robot-yaw-object-study-2026-10-04 (Autodesk Fusion 360 design; units mm, degrees)
Autodesk Fusion 360 part; units mm, degrees
sketch "Layout_Side" plane through (0, 0, 0) normal (0, 1, 0) x (1, 0, 0) in component "00_Layout"
  line L0 (0, 0) -> (0, -1676.4) construction
  line L1 (300, -275) -> (-300, -275) construction
  line L2 (-300, -275) -> (-300, -75) construction
  line L3 (-300, -75) -> (300, -75) construction
  line L4 (300, -75) -> (300, -275) construction
  line L5 (300, -275) -> (-300, -75) construction
  line L6 (-300, -275) -> (300, -75) construction
  line L7 (0, -1676.4) -> (600, -1676.4) construction
  line L8 (0, -175) -> (0, -75) construction
  dimension "d1" = 200
  dimension "d2" = 600
  dimension "d4" = 600
  dimension "d5" = 75
  dimension "d6" = 1676.4
  constraint vertical L0
  constraint horizontal L1
  constraint perpendicular L1 L2
  constraint parallel L1 L3
  constraint parallel L2 L4
  constraint perpendicular L0 L7
  constraint midpoint L3 L8.end
  constraint coincident L0.start origin
  constraint midpoint L8.start L5
  measures "d1" distance of L1.end L2.end
  measures "d2" distance of L1.start L1.end
  measures "d4" distance of L0.end L7.end
  measures "d5" distance of L0.start L8.end
  measures "d6" distance of L0.end L0.start
sketch "Base_Profile" plane through (0, 0, 0) normal (0, 1, 0) x (1, 0, 0) in component "01_Base_Envelope"
  line L0 (300, -275) -> (-300, -275)
  line L1 (-300, -275) -> (-300, -75)
  line L2 (-300, -75) -> (300, -75)
  line L3 (300, -75) -> (300, -275)
extrude "Chassis_Width_450mm" add sketch "Base_Profile" along normal mid plane 450 makes body 1 in component "01_Base_Envelope"
sketch "Mast_Envelope_Side_Profile" plane through (0, 0, 0) normal (0, 1, 0) x (1, 0, 0) in component "02_Mast_Envelope"
  line L0 (-160, -275) -> (-40, -275)
  line L1 (-40, -275) -> (-40, -1600)
  line L2 (-40, -1600) -> (-160, -1600)
  line L3 (-160, -1600) -> (-160, -275)
  line L4 (300, -275) -> (-300, -275) construction
  dimension "d9" = 120
  dimension "d10" = 1325
  dimension "d11" = 160
  constraint horizontal L0
  constraint vertical L1
  constraint horizontal L2
  constraint vertical L3
  constraint coincident L0.start L4
  measures "d9" horizontal distance of L0.start L0.end
  measures "d10" vertical distance of L0.end L1.end
  measures "d11" horizontal distance of origin L0.start
extrude "Mast_Envelope_Width_140mm" add sketch "Mast_Envelope_Side_Profile" along normal mid plane 140 separate body makes body 2 in component "02_Mast_Envelope"
sketch "Shared_Carriage_Side_Profile" plane through (0, 0, 0) normal (0, 1, 0) x (1, 0, 0) in component "03_Shared_Carriage"
  line L0 (-40, -840) -> (80, -840)
  line L1 (80, -840) -> (80, -960)
  line L2 (80, -960) -> (-40, -960)
  line L3 (-40, -960) -> (-40, -840)
  dimension "d14" = 120
  dimension "d15" = 120
  dimension "d16" = 40
  dimension "d17" = 840
  constraint horizontal L0
  constraint vertical L1
  constraint horizontal L2
  constraint vertical L3
  measures "d14" horizontal distance of L0.start L0.end
  measures "d15" vertical distance of L0.end L1.end
  measures "d16" horizontal distance of origin L0.start
  measures "d17" vertical distance of origin L0.start
extrude "Shared_Carriage_Width_660mm" add sketch "Shared_Carriage_Side_Profile" along normal mid plane 660 separate body makes body 3 in component "03_Shared_Carriage"
ref_plane "WorkPlane1" through (0, 300, 0) normal (0, 1, 0) x (0, 0, 1) in component "00_Layout"
sketch "Reach_Left_Floor_2x304p8mm" plane through (0, 300, 0) normal (0, 1, 0) x (1, 0, 0) in component "00_Layout"
  circle A0 centre (80, -400) radius 609.6 construction
  line L0 (80, -400) -> (380.0994, -346.6765) construction
  line L1 (380.0994, -346.6765) -> (450, -50) construction
  dimension "d25" = 80
  dimension "d26" = 400
  dimension "d27" = 450
  dimension "d28" = 50
  dimension "d29" = 609.6
  dimension "d30" = 304.8
  dimension "d31" = 304.8
  measures "d25" horizontal distance of origin A0.centre
  measures "d26" vertical distance of origin A0.centre
  measures "d27" horizontal distance of origin L1.end
  measures "d28" vertical distance of origin L1.end
  measures "d29" radius of A0
  measures "d30" distance of A0.centre L0.end
  measures "d31" distance of L1.end L0.end
sketch "Reach_Left_Shelf_2x304p8mm" plane through (0, 300, 0) normal (0, 1, 0) x (1, 0, 0) in component "00_Layout"
  circle A0 centre (80, -1400) radius 609.6 construction
  line L0 (80, -1400) -> (198.6357, -1680.7643) construction
  line L1 (198.6357, -1680.7643) -> (500, -1726.4) construction
  dimension "d32" = 80
  dimension "d33" = 1400
  dimension "d34" = 500
  dimension "d35" = 1726.4
  dimension "d36" = 609.6
  dimension "d37" = 304.8
  dimension "d38" = 304.8
  measures "d32" horizontal distance of origin A0.centre
  measures "d33" vertical distance of origin A0.centre
  measures "d34" horizontal distance of origin L1.end
  measures "d35" vertical distance of origin L1.end
  measures "d36" radius of A0
  measures "d37" distance of A0.centre L0.end
  measures "d38" distance of L1.end L0.end
ref_plane "WorkPlane2" through (0, -300, 0) normal (0, 1, 0) x (0, 0, 1) in component "00_Layout"
sketch "Reach_Right_Floor_2x304p8mm" plane through (0, -300, 0) normal (0, 1, 0) x (1, 0, 0) in component "00_Layout"
  circle A0 centre (80, -400) radius 609.6 construction
  line L0 (80, -400) -> (380.0994, -346.6765) construction
  line L1 (380.0994, -346.6765) -> (450, -50) construction
  dimension "d41" = 80
  dimension "d42" = 400
  dimension "d43" = 450
  dimension "d44" = 50
  dimension "d45" = 609.6
  dimension "d46" = 304.8
  dimension "d47" = 304.8
  measures "d41" horizontal distance of origin A0.centre
  measures "d42" vertical distance of origin A0.centre
  measures "d43" horizontal distance of origin L1.end
  measures "d44" vertical distance of origin L1.end
  measures "d45" radius of A0
  measures "d46" distance of A0.centre L0.end
  measures "d47" distance of L1.end L0.end
sketch "Reach_Right_Shelf_2x304p8mm" plane through (0, -300, 0) normal (0, 1, 0) x (1, 0, 0) in component "00_Layout"
  circle A0 centre (80, -1400) radius 609.6 construction
  line L0 (80, -1400) -> (198.6357, -1680.7643) construction
  line L1 (198.6357, -1680.7643) -> (500, -1726.4) construction
  dimension "d48" = 80
  dimension "d49" = 1400
  dimension "d50" = 500
  dimension "d51" = 1726.4
  dimension "d52" = 609.6
  dimension "d53" = 304.8
  dimension "d54" = 304.8
  measures "d48" horizontal distance of origin A0.centre
  measures "d49" vertical distance of origin A0.centre
  measures "d50" horizontal distance of origin L1.end
  measures "d51" vertical distance of origin L1.end
  measures "d52" radius of A0
  measures "d53" distance of A0.centre L0.end
  measures "d54" distance of L1.end L0.end
sketch "Shoulder_Mount_Profile" plane through (0, 0, 0) normal (0, 1, 0) x (1, 0, 0) in component "04_Left_Shoulder_Standoff"
  line L0 (-20, 20) -> (20, 20)
  line L1 (20, 20) -> (20, -20)
  line L2 (20, -20) -> (-20, -20)
  line L3 (-20, -20) -> (-20, 20)
  dimension "d55" = 20
  dimension "d56" = 20
  dimension "d57" = 40
  dimension "d58" = 40
  constraint horizontal L0
  constraint vertical L1
  constraint horizontal L2
  constraint vertical L3
  measures "d55" horizontal distance of origin L0.start
  measures "d56" vertical distance of origin L0.start
  measures "d57" horizontal distance of L0.start L0.end
  measures "d58" vertical distance of L0.end L1.end
extrude "Shoulder_Mount" add sketch "Shoulder_Mount_Profile" along normal mid plane 40 separate body makes body 4 in component "04_Left_Shoulder_Standoff"
sketch "Upper_Link_304p8mm_Profile" plane through (0, 0, 0) normal (0, 1, 0) x (1, 0, 0) in component "05_Left_Upper_Arm"
  line L0 (20, 20) -> (284.8, 20)
  line L1 (284.8, 20) -> (284.8, -20)
  line L2 (284.8, -20) -> (20, -20)
  line L3 (20, -20) -> (20, 20)
  dimension "d61" = 20
  dimension "d62" = 20
  dimension "d63" = 264.8
  dimension "d64" = 40
  constraint horizontal L0
  constraint vertical L1
  constraint horizontal L2
  constraint vertical L3
  measures "d61" horizontal distance of origin L0.start
  measures "d62" vertical distance of origin L0.start
  measures "d63" horizontal distance of L0.start L0.end
  measures "d64" vertical distance of L0.end L1.end
extrude "Upper_Link_304p8mm" add sketch "Upper_Link_304p8mm_Profile" along normal mid plane 24 separate body makes body 5 in component "05_Left_Upper_Arm"
sketch "Joint_Axis_Locations" plane through (0, 0, 0) normal (0, 1, 0) x (1, 0, 0) in component "05_Left_Upper_Arm"
  line L0 (0, 0) -> (304.8, 0) construction
  dimension "d67" = 304.8
  constraint horizontal L0
  measures "d67" horizontal distance of L0.start L0.end
sketch "Fore_Link_304p8mm_Profile" plane through (0, 0, 0) normal (0, 1, 0) x (1, 0, 0) in component "06_Left_Forearm"
  line L0 (20, 20) -> (284.8, 20)
  line L1 (284.8, 20) -> (284.8, -20)
  line L2 (284.8, -20) -> (20, -20)
  line L3 (20, -20) -> (20, 20)
  dimension "d68" = 20
  dimension "d69" = 20
  dimension "d70" = 264.8
  dimension "d71" = 40
  constraint horizontal L0
  constraint vertical L1
  constraint horizontal L2
  constraint vertical L3
  measures "d68" horizontal distance of origin L0.start
  measures "d69" vertical distance of origin L0.start
  measures "d70" horizontal distance of L0.start L0.end
  measures "d71" vertical distance of L0.end L1.end
extrude "Fore_Link_304p8mm" add sketch "Fore_Link_304p8mm_Profile" along normal mid plane 24 separate body makes body 6 in component "06_Left_Forearm"
sketch "Joint_Axis_Locations (2)" plane through (0, 0, 0) normal (0, 1, 0) x (1, 0, 0) in component "06_Left_Forearm"
  line L0 (0, 0) -> (304.8, 0) construction
  dimension "d74" = 304.8
  constraint horizontal L0
  measures "d74" horizontal distance of L0.start L0.end
sketch "Palm_Envelope_Profile" plane through (0, 0, 0) normal (0, 1, 0) x (1, 0, 0) in component "07_Left_Wrist_Palm"
  line L0 (5, 15) -> (60, 15)
  line L1 (60, 15) -> (60, -15)
  line L2 (60, -15) -> (5, -15)
  line L3 (5, -15) -> (5, 15)
  dimension "d75" = 5
  dimension "d76" = 15
  dimension "d77" = 55
  dimension "d78" = 30
  constraint horizontal L0
  constraint vertical L1
  constraint horizontal L2
  constraint vertical L3
  measures "d75" horizontal distance of origin L0.start
  measures "d76" vertical distance of origin L0.start
  measures "d77" horizontal distance of L0.start L0.end
  measures "d78" vertical distance of L0.end L1.end
extrude "Palm_Envelope" add sketch "Palm_Envelope_Profile" along normal mid plane 80 separate body makes body 7 in component "07_Left_Wrist_Palm"
sketch "Joint_Axis_Locations (3)" plane through (0, 0, 0) normal (0, 1, 0) x (1, 0, 0) in component "07_Left_Wrist_Palm"
  line L0 (0, 0) -> (110, 0) construction
  dimension "d81" = 110
  constraint horizontal L0
  measures "d81" horizontal distance of L0.start L0.end
sketch "Finger_Envelope_Profile" plane through (0, 0, 0) normal (0, 1, 0) x (1, 0, 0) in component "08_Left_Finger_Positive"
  line L0 (62, 15) -> (140, 15)
  line L1 (140, 15) -> (140, -15)
  line L2 (140, -15) -> (62, -15)
  line L3 (62, -15) -> (62, 15)
  dimension "d88" = 62
  dimension "d89" = 15
  dimension "d90" = 78
  dimension "d91" = 30
  constraint horizontal L0
  constraint vertical L1
  constraint horizontal L2
  constraint vertical L3
  measures "d88" horizontal distance of origin L0.start
  measures "d89" vertical distance of origin L0.start
  measures "d90" horizontal distance of L0.start L0.end
  measures "d91" vertical distance of L0.end L1.end
extrude "Finger_Envelope" add sketch "Finger_Envelope_Profile" along normal mid plane 10 separate body makes body 8 in component "08_Left_Finger_Positive"
sketch "Soft_Pad_Envelope_Profile" plane through (0, 0, 0) normal (0, 1, 0) x (1, 0, 0) in component "09_Left_Pad_Positive"
  line L0 (80, 14) -> (140, 14)
  line L1 (140, 14) -> (140, -14)
  line L2 (140, -14) -> (80, -14)
  line L3 (80, -14) -> (80, 14)
  dimension "d94" = 80
  dimension "d95" = 14
  dimension "d96" = 60
  dimension "d97" = 28
  constraint horizontal L0
  constraint vertical L1
  constraint horizontal L2
  constraint vertical L3
  measures "d94" horizontal distance of origin L0.start
  measures "d95" vertical distance of origin L0.start
  measures "d96" horizontal distance of L0.start L0.end
  measures "d97" vertical distance of L0.end L1.end
extrude "Soft_Pad_Envelope" add sketch "Soft_Pad_Envelope_Profile" along normal mid plane 3 separate body makes body 9 in component "09_Left_Pad_Positive"
sketch "Finger_Envelope_Profile (2)" plane through (0, 0, 0) normal (0, 1, 0) x (1, 0, 0) in component "08_Left_Finger_Negative"
  line L0 (62, 15) -> (140, 15)
  line L1 (140, 15) -> (140, -15)
  line L2 (140, -15) -> (62, -15)
  line L3 (62, -15) -> (62, 15)
  dimension "d102" = 62
  dimension "d103" = 15
  dimension "d104" = 78
  dimension "d105" = 30
  constraint horizontal L0
  constraint vertical L1
  constraint horizontal L2
  constraint vertical L3
  measures "d102" horizontal distance of origin L0.start
  measures "d103" vertical distance of origin L0.start
  measures "d104" horizontal distance of L0.start L0.end
  measures "d105" vertical distance of L0.end L1.end
extrude "Finger_Envelope'" add sketch "Finger_Envelope_Profile (2)" along normal mid plane 10 separate body makes body 10 in component "08_Left_Finger_Negative"
sketch "Soft_Pad_Envelope_Profile (2)" plane through (0, 0, 0) normal (0, 1, 0) x (1, 0, 0) in component "09_Left_Pad_Negative"
  line L0 (80, 14) -> (140, 14)
  line L1 (140, 14) -> (140, -14)
  line L2 (140, -14) -> (80, -14)
  line L3 (80, -14) -> (80, 14)
  dimension "d108" = 80
  dimension "d109" = 14
  dimension "d110" = 60
  dimension "d111" = 28
  constraint horizontal L0
  constraint vertical L1
  constraint horizontal L2
  constraint vertical L3
  measures "d108" horizontal distance of origin L0.start
  measures "d109" vertical distance of origin L0.start
  measures "d110" horizontal distance of L0.start L0.end
  measures "d111" vertical distance of L0.end L1.end
extrude "Soft_Pad_Envelope'" add sketch "Soft_Pad_Envelope_Profile (2)" along normal mid plane 3 separate body makes body 11 in component "09_Left_Pad_Negative"
sketch "Shoulder_Mount_Profile (2)" plane through (0, 0, 0) normal (0, 1, 0) x (1, 0, 0) in component "04_Right_Shoulder_Standoff"
  line L0 (-20, 20) -> (20, 20)
  line L1 (20, 20) -> (20, -20)
  line L2 (20, -20) -> (-20, -20)
  line L3 (-20, -20) -> (-20, 20)
  dimension "d116" = 20
  dimension "d117" = 20
  dimension "d118" = 40
  dimension "d119" = 40
  constraint horizontal L0
  constraint vertical L1
  constraint horizontal L2
  constraint vertical L3
  measures "d116" horizontal distance of origin L0.start
  measures "d117" vertical distance of origin L0.start
  measures "d118" horizontal distance of L0.start L0.end
  measures "d119" vertical distance of L0.end L1.end
extrude "Shoulder_Mount'" add sketch "Shoulder_Mount_Profile (2)" along normal mid plane 40 separate body makes body 12 in component "04_Right_Shoulder_Standoff"
sketch "Upper_Link_304p8mm_Profile (2)" plane through (0, 0, 0) normal (0, 1, 0) x (1, 0, 0) in component "05_Right_Upper_Arm"
  line L0 (20, 20) -> (284.8, 20)
  line L1 (284.8, 20) -> (284.8, -20)
  line L2 (284.8, -20) -> (20, -20)
  line L3 (20, -20) -> (20, 20)
  dimension "d122" = 20
  dimension "d123" = 20
  dimension "d124" = 264.8
  dimension "d125" = 40
  constraint horizontal L0
  constraint vertical L1
  constraint horizontal L2
  constraint vertical L3
  measures "d122" horizontal distance of origin L0.start
  measures "d123" vertical distance of origin L0.start
  measures "d124" horizontal distance of L0.start L0.end
  measures "d125" vertical distance of L0.end L1.end
extrude "Upper_Link_304p8mm'" add sketch "Upper_Link_304p8mm_Profile (2)" along normal mid plane 24 separate body makes body 13 in component "05_Right_Upper_Arm"
sketch "Joint_Axis_Locations (4)" plane through (0, 0, 0) normal (0, 1, 0) x (1, 0, 0) in component "05_Right_Upper_Arm"
  line L0 (0, 0) -> (304.8, 0) construction
  dimension "d128" = 304.8
  constraint horizontal L0
  measures "d128" horizontal distance of L0.start L0.end
sketch "Fore_Link_304p8mm_Profile (2)" plane through (0, 0, 0) normal (0, 1, 0) x (1, 0, 0) in component "06_Right_Forearm"
  line L0 (20, 20) -> (284.8, 20)
  line L1 (284.8, 20) -> (284.8, -20)
  line L2 (284.8, -20) -> (20, -20)
  line L3 (20, -20) -> (20, 20)
  dimension "d129" = 20
  dimension "d130" = 20
  dimension "d131" = 264.8
  dimension "d132" = 40
  constraint horizontal L0
  constraint vertical L1
  constraint horizontal L2
  constraint vertical L3
  measures "d129" horizontal distance of origin L0.start
  measures "d130" vertical distance of origin L0.start
  measures "d131" horizontal distance of L0.start L0.end
  measures "d132" vertical distance of L0.end L1.end
extrude "Fore_Link_304p8mm'" add sketch "Fore_Link_304p8mm_Profile (2)" along normal mid plane 24 separate body makes body 14 in component "06_Right_Forearm"
sketch "Joint_Axis_Locations (5)" plane through (0, 0, 0) normal (0, 1, 0) x (1, 0, 0) in component "06_Right_Forearm"
  line L0 (0, 0) -> (304.8, 0) construction
  dimension "d135" = 304.8
  constraint horizontal L0
  measures "d135" horizontal distance of L0.start L0.end
sketch "Palm_Envelope_Profile (2)" plane through (0, 0, 0) normal (0, 1, 0) x (1, 0, 0) in component "07_Right_Wrist_Palm"
  line L0 (5, 15) -> (60, 15)
  line L1 (60, 15) -> (60, -15)
  line L2 (60, -15) -> (5, -15)
  line L3 (5, -15) -> (5, 15)
  dimension "d136" = 5
  dimension "d137" = 15
  dimension "d138" = 55
  dimension "d139" = 30
  constraint horizontal L0
  constraint vertical L1
  constraint horizontal L2
  constraint vertical L3
  measures "d136" horizontal distance of origin L0.start
  measures "d137" vertical distance of origin L0.start
  measures "d138" horizontal distance of L0.start L0.end
  measures "d139" vertical distance of L0.end L1.end
extrude "Palm_Envelope'" add sketch "Palm_Envelope_Profile (2)" along normal mid plane 80 separate body makes body 15 in component "07_Right_Wrist_Palm"
sketch "Joint_Axis_Locations (6)" plane through (0, 0, 0) normal (0, 1, 0) x (1, 0, 0) in component "07_Right_Wrist_Palm"
  line L0 (0, 0) -> (110, 0) construction
  dimension "d142" = 110
  constraint horizontal L0
  measures "d142" horizontal distance of L0.start L0.end
sketch "Finger_Envelope_Profile (3)" plane through (0, 0, 0) normal (0, 1, 0) x (1, 0, 0) in component "08_Right_Finger_Positive"
  line L0 (62, 15) -> (140, 15)
  line L1 (140, 15) -> (140, -15)
  line L2 (140, -15) -> (62, -15)
  line L3 (62, -15) -> (62, 15)
  dimension "d149" = 62
  dimension "d150" = 15
  dimension "d151" = 78
  dimension "d152" = 30
  constraint horizontal L0
  constraint vertical L1
  constraint horizontal L2
  constraint vertical L3
  measures "d149" horizontal distance of origin L0.start
  measures "d150" vertical distance of origin L0.start
  measures "d151" horizontal distance of L0.start L0.end
  measures "d152" vertical distance of L0.end L1.end
extrude "Finger_Envelope''" add sketch "Finger_Envelope_Profile (3)" along normal mid plane 10 separate body makes body 16 in component "08_Right_Finger_Positive"
sketch "Soft_Pad_Envelope_Profile (3)" plane through (0, 0, 0) normal (0, 1, 0) x (1, 0, 0) in component "09_Right_Pad_Positive"
  line L0 (80, 14) -> (140, 14)
  line L1 (140, 14) -> (140, -14)
  line L2 (140, -14) -> (80, -14)
  line L3 (80, -14) -> (80, 14)
  dimension "d155" = 80
  dimension "d156" = 14
  dimension "d157" = 60
  dimension "d158" = 28
  constraint horizontal L0
  constraint vertical L1
  constraint horizontal L2
  constraint vertical L3
  measures "d155" horizontal distance of origin L0.start
  measures "d156" vertical distance of origin L0.start
  measures "d157" horizontal distance of L0.start L0.end
  measures "d158" vertical distance of L0.end L1.end
extrude "Soft_Pad_Envelope''" add sketch "Soft_Pad_Envelope_Profile (3)" along normal mid plane 3 separate body makes body 17 in component "09_Right_Pad_Positive"
sketch "Finger_Envelope_Profile (4)" plane through (0, 0, 0) normal (0, 1, 0) x (1, 0, 0) in component "08_Right_Finger_Negative"
  line L0 (62, 15) -> (140, 15)
  line L1 (140, 15) -> (140, -15)
  line L2 (140, -15) -> (62, -15)
  line L3 (62, -15) -> (62, 15)
  dimension "d163" = 62
  dimension "d164" = 15
  dimension "d165" = 78
  dimension "d166" = 30
  constraint horizontal L0
  constraint vertical L1
  constraint horizontal L2
  constraint vertical L3
  measures "d163" horizontal distance of origin L0.start
  measures "d164" vertical distance of origin L0.start
  measures "d165" horizontal distance of L0.start L0.end
  measures "d166" vertical distance of L0.end L1.end
extrude "Finger_Envelope'''" add sketch "Finger_Envelope_Profile (4)" along normal mid plane 10 separate body makes body 18 in component "08_Right_Finger_Negative"
sketch "Soft_Pad_Envelope_Profile (4)" plane through (0, 0, 0) normal (0, 1, 0) x (1, 0, 0) in component "09_Right_Pad_Negative"
  line L0 (80, 14) -> (140, 14)
  line L1 (140, 14) -> (140, -14)
  line L2 (140, -14) -> (80, -14)
  line L3 (80, -14) -> (80, 14)
  dimension "d169" = 80
  dimension "d170" = 14
  dimension "d171" = 60
  dimension "d172" = 28
  constraint horizontal L0
  constraint vertical L1
  constraint horizontal L2
  constraint vertical L3
  measures "d169" horizontal distance of origin L0.start
  measures "d170" vertical distance of origin L0.start
  measures "d171" horizontal distance of L0.start L0.end
  measures "d172" vertical distance of L0.end L1.end
extrude "Soft_Pad_Envelope'''" add sketch "Soft_Pad_Envelope_Profile (4)" along normal mid plane 3 separate body makes body 19 in component "09_Right_Pad_Negative"
sketch "Pivot_Housing_Envelopes" plane through (0, 0, 0) normal (0, 1, 0) x (1, 0, 0) in component "05_Left_Upper_Arm"
  circle A0 centre (0, 0) radius 25
  line L0 (0, 0) -> (304.8, 0) construction
  circle A1 centre (304.8, 0) radius 25
  dimension "d177" = 25
  dimension "d178" = 304.8
  dimension "d179" = 25
  constraint coincident A0.centre L0.start
  constraint horizontal L0
  measures "d177" radius of A0
  measures "d178" horizontal distance of A0.centre L0.end
  measures "d179" radius of A1
extrude "Pivot_Housing_Envelopes_24mm" add sketch "Pivot_Housing_Envelopes" along normal mid plane 24 bodies 5 in component "05_Left_Upper_Arm"
sketch "Pivot_Housing_Envelopes (2)" plane through (0, 0, 0) normal (0, 1, 0) x (1, 0, 0) in component "06_Left_Forearm"
  circle A0 centre (0, 0) radius 25
  line L0 (0, 0) -> (304.8, 0) construction
  circle A1 centre (304.8, 0) radius 25
  dimension "d182" = 25
  dimension "d183" = 304.8
  dimension "d184" = 25
  constraint coincident A0.centre L0.start
  constraint horizontal L0
  measures "d182" radius of A0
  measures "d183" horizontal distance of A0.centre L0.end
  measures "d184" radius of A1
extrude "Pivot_Housing_Envelopes_24mm'" add sketch "Pivot_Housing_Envelopes (2)" along normal mid plane 24 bodies 6 in component "06_Left_Forearm"
sketch "Pivot_Housing_Envelopes (3)" plane through (0, 0, 0) normal (0, 1, 0) x (1, 0, 0) in component "05_Right_Upper_Arm"
  circle A0 centre (0, 0) radius 25
  line L0 (0, 0) -> (304.8, 0) construction
  circle A1 centre (304.8, 0) radius 25
  dimension "d187" = 25
  dimension "d188" = 304.8
  dimension "d189" = 25
  constraint coincident A0.centre L0.start
  constraint horizontal L0
  measures "d187" radius of A0
  measures "d188" horizontal distance of A0.centre L0.end
  measures "d189" radius of A1
extrude "Pivot_Housing_Envelopes_24mm''" add sketch "Pivot_Housing_Envelopes (3)" along normal mid plane 24 bodies 13 in component "05_Right_Upper_Arm"
sketch "Pivot_Housing_Envelopes (4)" plane through (0, 0, 0) normal (0, 1, 0) x (1, 0, 0) in component "06_Right_Forearm"
  circle A0 centre (0, 0) radius 25
  line L0 (0, 0) -> (304.8, 0) construction
  circle A1 centre (304.8, 0) radius 25
  dimension "d192" = 25
  dimension "d193" = 304.8
  dimension "d194" = 25
  constraint coincident A0.centre L0.start
  constraint horizontal L0
  measures "d192" radius of A0
  measures "d193" horizontal distance of A0.centre L0.end
  measures "d194" radius of A1
extrude "Pivot_Housing_Envelopes_24mm'''" add sketch "Pivot_Housing_Envelopes (4)" along normal mid plane 24 bodies 14 in component "06_Right_Forearm"
sketch "Shoulder_Pitch_Sweep_Clearance_35p5mm" plane through (0, 0, 0) normal (0, 1, 0) x (1, 0, 0) in component "04_Left_Shoulder_Standoff"
  line L0 (0, 0) -> (20, 0) construction
  circle A0 centre (20, 0) radius 35.5
  dimension "d197" = 20
  dimension "d198" = 35.5
  constraint horizontal L0
  measures "d197" horizontal distance of L0.start L0.end
  measures "d198" radius of A0
sketch "Wrist_Sweep_Clearance_35p5mm" plane through (0, 0, 0) normal (0, 1, 0) x (1, 0, 0) in component "07_Left_Wrist_Palm"
  circle A0 centre (0, 0) radius 35.5
  dimension "d203" = 35.5
  measures "d203" radius of A0
sketch "Shoulder_Pitch_Sweep_Clearance_35p5mm (2)" plane through (0, 0, 0) normal (0, 1, 0) x (1, 0, 0) in component "04_Right_Shoulder_Standoff"
  line L0 (0, 0) -> (20, 0) construction
  circle A0 centre (20, 0) radius 35.5
  dimension "d208" = 20
  dimension "d209" = 35.5
  constraint horizontal L0
  measures "d208" horizontal distance of L0.start L0.end
  measures "d209" radius of A0
sketch "Wrist_Sweep_Clearance_35p5mm (2)" plane through (0, 0, 0) normal (0, 1, 0) x (1, 0, 0) in component "07_Right_Wrist_Palm"
  circle A0 centre (0, 0) radius 35.5
  dimension "d214" = 35.5
  measures "d214" radius of A0
extrude "Pivot_Clearance_Cut_This_Component_Only" cut sketch "Shoulder_Pitch_Sweep_Clearance_35p5mm" along normal mid plane 90 bodies 4 in component "04_Left_Shoulder_Standoff"
extrude "Pivot_Clearance_Cut_This_Component_Only'" cut sketch "Wrist_Sweep_Clearance_35p5mm" along normal mid plane 90 bodies 7 in component "07_Left_Wrist_Palm"
extrude "Pivot_Clearance_Cut_This_Component_Only''" cut sketch "Shoulder_Pitch_Sweep_Clearance_35p5mm (2)" along normal mid plane 90 bodies 12 in component "04_Right_Shoulder_Standoff"
extrude "Pivot_Clearance_Cut_This_Component_Only'''" cut sketch "Wrist_Sweep_Clearance_35p5mm (2)" along normal mid plane 90 bodies 15 in component "07_Right_Wrist_Palm"
sketch "Yaw_Axis_XY_Location" plane through (0, 0, 0) normal (0, 0, 1) x (1, 0, 0) in component "04_Left_Shoulder_Standoff"
  line L0 (0, 0) -> (20, 0) construction
  dimension "d262" = 20
  constraint horizontal L0
  measures "d262" horizontal distance of L0.start L0.end
sketch "Yaw_Axis_XY_Location (2)" plane through (0, 0, 0) normal (0, 0, 1) x (1, 0, 0) in component "04_Right_Shoulder_Standoff"
  line L0 (0, 0) -> (20, 0) construction
  dimension "d265" = 20
  constraint horizontal L0
  measures "d265" horizontal distance of L0.start L0.end
ref_plane "WorkPlane1" through (0, 0, 840) normal (0, 0, 1) x (1, 0, 0) in component "03_Shared_Carriage"
sketch "Shoulder_Yaw_Sweep_Relief_30" plane through (0, 0, 840) normal (0, 0, 1) x (1, 0, 0) in component "03_Shared_Carriage"
  line L0 (0, 0) -> (120, 300) construction
  circle A0 centre (120, 300) radius 50.5
  dimension "d270" = 120
  dimension "d271" = 300
  dimension "d272" = 50.5
  measures "d270" horizontal distance of L0.start L0.end
  measures "d271" vertical distance of L0.start L0.end
  measures "d272" radius of A0
extrude "Yaw_Sweep_Clearance_Carriage_Only" cut sketch "Shoulder_Yaw_Sweep_Relief_30" along normal blind 120 bodies 3 in component "03_Shared_Carriage"
ref_plane "WorkPlane2" through (0, 0, 840) normal (0, 0, 1) x (1, 0, 0) in component "03_Shared_Carriage"
sketch "Shoulder_Yaw_Sweep_Relief_-30" plane through (0, 0, 840) normal (0, 0, 1) x (1, 0, 0) in component "03_Shared_Carriage"
  line L0 (0, 0) -> (120, -300) construction
  circle A0 centre (120, -300) radius 50.5
  dimension "d277" = 120
  dimension "d278" = 300
  dimension "d279" = 50.5
  measures "d277" horizontal distance of L0.start L0.end
  measures "d278" vertical distance of L0.start L0.end
  measures "d279" radius of A0
extrude "Yaw_Sweep_Clearance_Carriage_Only (1)" cut sketch "Shoulder_Yaw_Sweep_Relief_-30" along normal blind 120 bodies 3 in component "03_Shared_Carriage"
ref_plane "WorkPlane1" through (0, 0, -60) normal (0, 0, 1) x (1, 0, 0) in component "04_Left_Shoulder_Standoff"
sketch "Yaw_Rotor_88mm_Envelope" plane through (0, 0, -60) normal (0, 0, 1) x (1, 0, 0) in component "04_Left_Shoulder_Standoff"
  line L0 (0, 0) -> (20, 0) construction
  circle A0 centre (20, 0) radius 44
  dimension "d284" = 20
  dimension "d285" = 44
  constraint horizontal L0
  measures "d284" horizontal distance of L0.start L0.end
  measures "d285" radius of A0
extrude "Left_Yaw_Rotor_Packaging" add sketch "Yaw_Rotor_88mm_Envelope" along normal blind 30 separate body makes body 20 in component "04_Left_Shoulder_Standoff"
ref_plane "WorkPlane1" through (0, 0, -60) normal (0, 0, 1) x (1, 0, 0) in component "04_Left_Yaw_Bearing_Housing"
sketch "Bearing_Housing_100mm_Envelope" plane through (0, 0, -60) normal (0, 0, 1) x (1, 0, 0) in component "04_Left_Yaw_Bearing_Housing"
  circle A0 centre (0, 0) radius 45.5
  circle A1 centre (0, 0) radius 50
  dimension "d290" = 45.5
  dimension "d291" = 50
  measures "d290" radius of A0
  measures "d291" radius of A1
extrude "Left_Yaw_Bearing_Housing_Packaging" add sketch "Bearing_Housing_100mm_Envelope" along normal blind 30 separate body makes body 21 in component "04_Left_Yaw_Bearing_Housing"
ref_plane "WorkPlane1" through (0, 0, -60) normal (0, 0, 1) x (1, 0, 0) in component "04_Right_Shoulder_Standoff"
sketch "Yaw_Rotor_88mm_Envelope (2)" plane through (0, 0, -60) normal (0, 0, 1) x (1, 0, 0) in component "04_Right_Shoulder_Standoff"
  line L0 (0, 0) -> (20, 0) construction
  circle A0 centre (20, 0) radius 44
  dimension "d296" = 20
  dimension "d297" = 44
  constraint horizontal L0
  measures "d296" horizontal distance of L0.start L0.end
  measures "d297" radius of A0
extrude "Right_Yaw_Rotor_Packaging" add sketch "Yaw_Rotor_88mm_Envelope (2)" along normal blind 30 separate body makes body 22 in component "04_Right_Shoulder_Standoff"
ref_plane "WorkPlane1" through (0, 0, -60) normal (0, 0, 1) x (1, 0, 0) in component "04_Right_Yaw_Bearing_Housing"
sketch "Bearing_Housing_100mm_Envelope (2)" plane through (0, 0, -60) normal (0, 0, 1) x (1, 0, 0) in component "04_Right_Yaw_Bearing_Housing"
  circle A0 centre (0, 0) radius 45.5
  circle A1 centre (0, 0) radius 50
  dimension "d302" = 45.5
  dimension "d303" = 50
  measures "d302" radius of A0
  measures "d303" radius of A1
extrude "Right_Yaw_Bearing_Housing_Packaging" add sketch "Bearing_Housing_100mm_Envelope (2)" along normal blind 30 separate body makes body 23 in component "04_Right_Yaw_Bearing_Housing"
sketch "ASSUMED_Pillow_Envelope_Profile" plane through (0, 0, 0) normal (0, 1, 0) x (1, 0, 0) in component "10_ASSUMED_Pillow_300x400x60mm"
  line L0 (-150, 30) -> (150, 30)
  line L1 (150, 30) -> (150, -30)
  line L2 (150, -30) -> (-150, -30)
  line L3 (-150, -30) -> (-150, 30)
  dimension "d306" = 150
  dimension "d307" = 30
  dimension "d308" = 300
  dimension "d309" = 60
  constraint horizontal L0
  constraint vertical L1
  constraint horizontal L2
  constraint vertical L3
  measures "d306" horizontal distance of origin L0.start
  measures "d307" vertical distance of origin L0.start
  measures "d308" horizontal distance of L0.start L0.end
  measures "d309" vertical distance of L0.end L1.end
extrude "ASSUMED_Pillow_Envelope" add sketch "ASSUMED_Pillow_Envelope_Profile" along normal mid plane 400 separate body makes body 24 in component "10_ASSUMED_Pillow_300x400x60mm"
sketch "ASSUMED_Box_Envelope_Profile" plane through (0, 0, 0) normal (0, 1, 0) x (1, 0, 0) in component "10_ASSUMED_Box_100x60x80mm"
  line L0 (-50, 40) -> (50, 40)
  line L1 (50, 40) -> (50, -40)
  line L2 (50, -40) -> (-50, -40)
  line L3 (-50, -40) -> (-50, 40)
  dimension "d312" = 50
  dimension "d313" = 40
  dimension "d314" = 100
  dimension "d315" = 80
  constraint horizontal L0
  constraint vertical L1
  constraint horizontal L2
  constraint vertical L3
  measures "d312" horizontal distance of origin L0.start
  measures "d313" vertical distance of origin L0.start
  measures "d314" horizontal distance of L0.start L0.end
  measures "d315" vertical distance of L0.end L1.end
extrude "ASSUMED_Box_Envelope" add sketch "ASSUMED_Box_Envelope_Profile" along normal mid plane 60 separate body makes body 25 in component "10_ASSUMED_Box_100x60x80mm"
sketch "ASSUMED_Bottle_Section" plane through (0, 0, 0) normal (0, 0, 1) x (1, 0, 0) in component "10_ASSUMED_Bottle_D60x220mm"
  circle A0 centre (0, 0) radius 30
  dimension "d318" = 30
  measures "d318" radius of A0
extrude "ASSUMED_Bottle_Envelope" add sketch "ASSUMED_Bottle_Section" along normal blind 220 separate body makes body 26 in component "10_ASSUMED_Bottle_D60x220mm"
sketch "ASSUMED_Shelf_Surface_1676p4mm_Profile" plane through (0, 0, 0) normal (0, 1, 0) x (1, 0, 0) in component "10_ASSUMED_Shelf_400x1000x25mm"
  line L0 (-200, 12.5) -> (200, 12.5)
  line L1 (200, 12.5) -> (200, -12.5)
  line L2 (200, -12.5) -> (-200, -12.5)
  line L3 (-200, -12.5) -> (-200, 12.5)
  dimension "d321" = 200
  dimension "d322" = 12.5
  dimension "d323" = 400
  dimension "d324" = 25
  constraint horizontal L0
  constraint vertical L1
  constraint horizontal L2
  constraint vertical L3
  measures "d321" horizontal distance of origin L0.start
  measures "d322" vertical distance of origin L0.start
  measures "d323" horizontal distance of L0.start L0.end
  measures "d324" vertical distance of L0.end L1.end
extrude "ASSUMED_Shelf_Surface_1676p4mm" add sketch "ASSUMED_Shelf_Surface_1676p4mm_Profile" along normal mid plane 1000 separate body makes body 27 in component "10_ASSUMED_Shelf_400x1000x25mm"
component "00_Layout" placed x (1, 0, 0) y (0, 1, 0) z (0, 0, 1) at (0, 0, 0)
component "01_Base_Envelope" placed x (1, 0, 0) y (0, 1, 0) z (0, 0, 1) at (0, 0, 0)
component "02_Mast_Envelope" placed x (1, 0, 0) y (0, 1, 0) z (0, 0, 1) at (0, 0, 0)
component "03_Shared_Carriage" placed x (1, 0, 0) y (0, 1, 0) z (0, 0, 1) at (0, 0, 0)
component "04_Left_Shoulder_Standoff" placed x (0.983255, -0.182236, 0) y (0.182236, 0.983255, 0) z (0, 0, 1) at (100.3349, 303.6447, 900)
component "05_Left_Upper_Arm" placed x (0.434113, -0.080458, 0.897258) y (0.182236, 0.983255, 0) z (-0.882234, 0.163512, 0.441506) at (120, 300, 900)
component "06_Left_Forearm" placed x (0.434113, -0.080458, -0.897258) y (0.182236, 0.983255, 0) z (0.882234, -0.163512, 0.441506) at (259.607, 314.8066, 1173.4844)
component "07_Left_Wrist_Palm" placed x (0.983255, -0.182236, 0) y (0.182236, 0.983255, 0) z (0, 0, 1) at (391.9246, 290.283, 900)
component "08_Left_Finger_Positive" placed x (0.983255, -0.182236, 0) y (0.182236, 0.983255, 0) z (0, 0, 1) at (402.4942, 347.3118, 900)
component "09_Left_Pad_Positive" placed x (0.983255, -0.182236, 0) y (0.182236, 0.983255, 0) z (0, 0, 1) at (401.3097, 340.9206, 900)
component "08_Left_Finger_Negative" placed x (0.983255, -0.182236, 0) y (0.182236, 0.983255, 0) z (0, 0, 1) at (381.3549, 233.2542, 900)
component "09_Left_Pad_Negative" placed x (0.983255, -0.182236, 0) y (0.182236, 0.983255, 0) z (0, 0, 1) at (382.5395, 239.6453, 900)
component "04_Right_Shoulder_Standoff" placed x (0.983255, 0.182236, 0) y (-0.182236, 0.983255, 0) z (0, 0, 1) at (100.3349, -303.6447, 900)
component "05_Right_Upper_Arm" placed x (0.434113, 0.080458, 0.897258) y (-0.182236, 0.983255, 0) z (-0.882234, -0.163512, 0.441506) at (120, -300, 900)
component "06_Right_Forearm" placed x (0.434113, 0.080458, -0.897258) y (-0.182236, 0.983255, 0) z (0.882234, 0.163512, 0.441506) at (259.607, -314.8066, 1173.4844)
component "07_Right_Wrist_Palm" placed x (0.983255, 0.182236, 0) y (-0.182236, 0.983255, 0) z (0, 0, 1) at (391.9246, -290.283, 900)
component "08_Right_Finger_Positive" placed x (0.983255, 0.182236, 0) y (-0.182236, 0.983255, 0) z (0, 0, 1) at (381.3549, -233.2542, 900)
component "09_Right_Pad_Positive" placed x (0.983255, 0.182236, 0) y (-0.182236, 0.983255, 0) z (0, 0, 1) at (382.5395, -239.6453, 900)
component "08_Right_Finger_Negative" placed x (0.983255, 0.182236, 0) y (-0.182236, 0.983255, 0) z (0, 0, 1) at (402.4942, -347.3118, 900)
component "09_Right_Pad_Negative" placed x (0.983255, 0.182236, 0) y (-0.182236, 0.983255, 0) z (0, 0, 1) at (401.3097, -340.9206, 900)
component "04_Left_Yaw_Bearing_Housing" placed x (1, 0, 0) y (0, 1, 0) z (0, 0, 1) at (120, 300, 900)
component "04_Right_Yaw_Bearing_Housing" placed x (1, 0, 0) y (0, 1, 0) z (0, 0, 1) at (120, -300, 900)
component "10_ASSUMED_Pillow_300x400x60mm" placed x (1, 0, 0) y (0, 1, 0) z (0, 0, 1) at (500, 0, 900)
component "10_ASSUMED_Box_100x60x80mm" placed x (1, 0, 0) y (0, 1, 0) z (0, 0, 1) at (471, 340, 1716.4)
component "10_ASSUMED_Bottle_D60x220mm" placed x (1, 0, 0) y (0, 1, 0) z (0, 0, 1) at (450, 0, 0)
component "10_ASSUMED_Shelf_400x1000x25mm" placed x (1, 0, 0) y (0, 1, 0) z (0, 0, 1) at (600, 0, 1663.9)
named bodies: "Chassis_Envelope", "Mast_Envelope_Packaging_Only", "Shared_Carriage_Packaging_Only", "Shoulder_Mount_Packaging", "Upper_Link_304p8mm_Packaging", "Fore_Link_304p8mm_Packaging", "Palm_Envelope_Packaging", "Finger_Envelope_Packaging", "Soft_Pad_Envelope_Packaging", "Left_Yaw_Rotor_Packaging", "Left_Yaw_Bearing_Housing_Packaging", "Right_Yaw_Rotor_Packaging", "Right_Yaw_Bearing_Housing_Packaging", "ASSUMED_Pillow_Envelope_Packaging", "ASSUMED_Box_Envelope_Packaging", "ASSUMED_Bottle_Envelope", "ASSUMED_Shelf_Surface_1676p4mm_Packaging"
